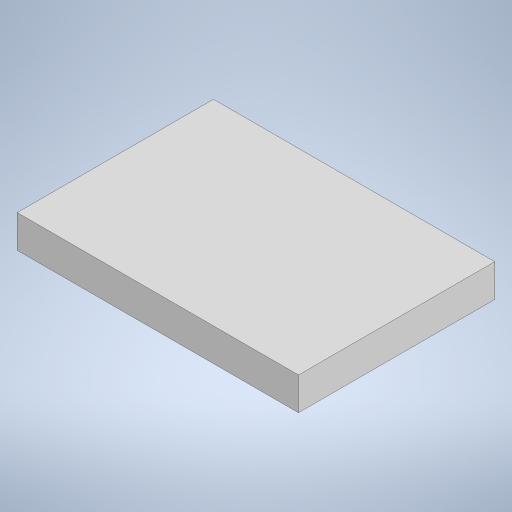
# Autodesk Inventor part: TestPlate
Saved by Autodesk Inventor 2023 (Build 270158030, 158C)
## iProperties
Created: 2022-06-08
Part Number: TestPlate
Material: Generic
Document SubType Name: Modeling
Designer: snobo
Density: 1 g/cm^3
Appearance: Default
Author: snobo
Autodesk Inventor part; units mm, degrees
ref_plane "YZ Plane" through (0, 0, 0) normal (1, 0, 0) x (0, 1, 0)
ref_plane "XZ Plane" through (0, 0, 0) normal (0, 1, 0) x (-1, 0, 0)
ref_plane "XY Plane" through (0, 0, 0) normal (0, 0, 1) x (1, 0, 0)
sketch "Sketch1" plane through (0, 0, 0) normal (0, 1, 0) x (-1, 0, 0)
  line L0 (107.5, 75) -> (-107.5, 75)
  line L1 (-107.5, 75) -> (-107.5, -75)
  line L2 (-107.5, -75) -> (107.5, -75)
  line L3 (107.5, -75) -> (107.5, 75)
  line L4 (107.5, 75) -> (-107.5, -75) construction
  line L5 (-107.5, 75) -> (107.5, -75) construction
  point P0 (0, 0)
  dimension "d0" = 215
  dimension "d1" = 150
  constraints: 12 end point, 2 midpoint, 2 parallel, 1 horizontal, 1 perpendicular
  measures "d0" distance of L1.end L2.end
  measures "d1" distance of L2.end L0.start
extrude "Extrusion1" add sketch "Sketch1" along normal blind 25
body "Solid1"
